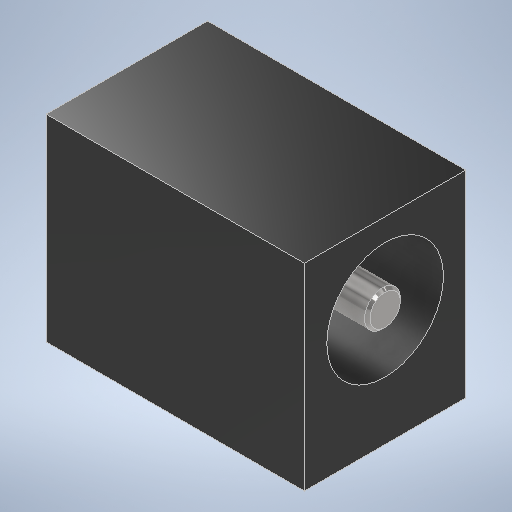
# Autodesk Inventor part: 9V_input
Saved by Autodesk Inventor 2025 (Build 290162000, 162)
## iProperties
Created: 2026-04-04
Part Number: 9V_input
Material: Polipropylen
Document SubType Name: Modeling
Designer: zzapa
Density: 0.899 g/cm^3
Appearance: Lśniąca — czarna
Author: zzapa
Autodesk Inventor part; units mm, degrees
ref_plane "YZ Plane" through (0, 0, 0) normal (1, 0, 0) x (0, 1, 0)
ref_plane "XZ Plane" through (0, 0, 0) normal (0, 1, 0) x (-1, 0, 0)
ref_plane "XY Plane" through (0, 0, 0) normal (0, 0, 1) x (1, 0, 0)
sketch "Szkic1" plane through (0, 0, 0) normal (0, 1, 0) x (-1, 0, 0)
  line L0 (14.4, -9) -> (0, -9)
  line L1 (0, -9) -> (0, 0)
  line L2 (0, 0) -> (14.4, 0)
  line L3 (14.4, 0) -> (14.4, -9)
  dimension "d0" = 9
  dimension "d1" = 14.4
  constraints: 8 end point, 2 parallel, 1 horizontal, 1 perpendicular
  measures "d0" distance of L2.end L0.start
  measures "d1" distance of L0.start L0.end
extrude "Wyciągnięcie proste1" add sketch "Szkic1" along normal blind 11
sketch "Szkic2" plane through (0, 0, 0) normal (1, 0, 0) x (0, 0, -1)
  line L0 (0, 11) -> (9, 11) projected
  line L1 (4.5, 11) -> (4.5, 0)
  line L2 (0, 0) -> (9, 0) projected
  circle A0 centre (4.5, 6.5) radius 1
  circle A1 centre (4.5, 6.5) radius 3.25
  dimension "d4" = 2
  dimension "d5" = 6.5
  dimension "d6" = 6.5
  constraints: 2 centre point, 2 end point, 2 midpoint, 1 coincident, 1 point on line
  measures "d4" diameter of A0
  measures "d5" diameter of A1
  measures "d6" distance from line of L2 A0.centre
extrude "Wyciągnięcie proste2" cut sketch "Szkic2" against normal blind 7 contours A1 L1 A0 | L1 A0 A1
chamfer "Faza1" distance 0.15 angle 45 1 edges at (0, 6.5, -3.5)
equation "\"d0\" = input_a"
equation "\"d1\" = input_b"
equation "\"d2\" = input_wys"
equation "\"gniazdo_M2_glebokosc\" = 1.5"
equation "\"gniazdo_M2_D1\" = 4.5"
equation "\"gniazdo_M2_D2\" = 2.6"
equation "\"insert_D\" = 2.4"
equation "\"insert_glebokosc\" = 5.5"
equation "\"podstawa_b\" = 65"
equation "\"podstawa_wys\" = 2"
equation "\"podstawa_otwory_montazowe_poz_x\" = 4"
equation "\"podstawa_otwory_montazowe_poz_y\" = 4"
equation "\"podstawa_zaokraglenie\" = 3"
equation "\"obudowa_b\" = 65"
equation "\"obudowa_wys\" = 36"
equation "\"obudowa_grubosc\" = 2"
equation "\"obudowa_kontrolki_a\" = 38"
equation "\"obudowa_otwory_montazowe_poz_x\" = 4"
equation "\"obudowa_otwory_montazowe_poz_y\" = 4"
equation "\"obudowa_otwory_montazowe_material_x\" = 8"
equation "\"obudowa_otwory_montazowe_material_y\" = 8"
equation "\"obudowa_zaokraglenie\" = 3"
equation "\"obudowa_otwory_io1_D\" = 11.5"
equation "\"obudowa_otwory_io1_wys\" = 15"
equation "\"obudowa_otwory_io2_D\" = 11.5"
equation "\"obudowa_otwory_io2_wys\" = 15"
equation "\"obudowa_otwory_pot_D\" = 8"
equation "\"input_a\" = 9"
equation "\"input_b\" = 14.4"
equation "\"input_wys\" = 11"
